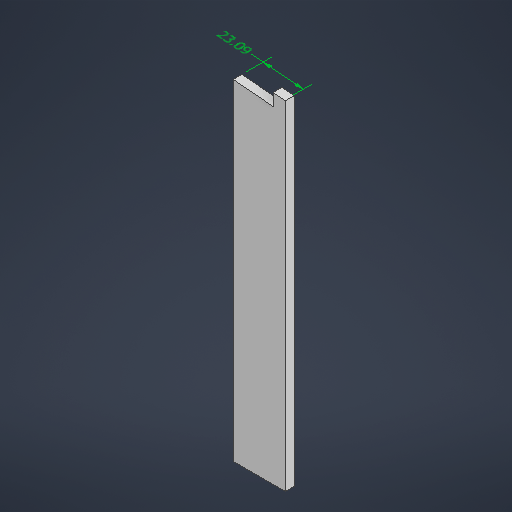
# Autodesk Inventor part: protostand
Saved by Autodesk Inventor 2026.2 (Build 302298000, 298)
## iProperties
Created: 2026-04-18
Part Number: protostand
Material: Generic
Document SubType Name: Modeling
Designer: danda
Density: 1 g/cm^3
Appearance: Default
Author: danda
Autodesk Inventor part; units mm, degrees
ref_plane "YZ Plane" through (0, 0, 0) normal (1, 0, 0) x (0, 1, 0)
ref_plane "XZ Plane" through (0, 0, 0) normal (0, 1, 0) x (-1, 0, 0)
ref_plane "XY Plane" through (0, 0, 0) normal (0, 0, 1) x (1, 0, 0)
sketch "Sketch1" plane through (0, 0, 0) normal (0, 0, 1) x (1, 0, 0)
  line L0 (65.4735, 181.5397) -> (65.4735, -8.4603)
  line L1 (65.4735, -8.4603) -> (95.4735, -8.4603)
  line L2 (95.4735, -8.4603) -> (95.4735, 178.9151)
  line L3 (65.4735, 181.5397) -> (95.4735, 178.9151)
  line L4 (65.4735, 181.5397) -> (99.7821, 181.5397) construction
  line L5 (95.4735, 178.9151) -> (95.4735, 186.5397)
  line L6 (95.4735, 186.5397) -> (88.4735, 186.5397)
  line L7 (88.4735, 186.5397) -> (88.4735, 179.5275)
  line L8 (88.4735, 186.5397) -> (98.471, 185.6651)
  line L9 (88.4735, 186.5397) -> (98.5092, 186.5397) construction
  point P0 (0, 0)
  point P1 (95.4735, 185.9273)
  dimension "d0" = 190
  dimension "d1" = 30
  dimension "d2" = 5
  dimension "d4" = 7
  dimension "d5" = 5
  dimension "d6" = 5
  constraints: 20 end point, 5 perpendicular, 2 horizontal, 1 equal length, 1 point on line, 1 vertical
  measures "d0" distance of L0.start L0.end
  measures "d1" distance of L0.end L1.end
  measures "d2" angle of L3 L4
  measures "d4" distance of L5.end L6.end
  measures "d5" distance between parallel lines of L6 L4
  measures "d6" angle of L8 L9
extrude "Extrusion1" add sketch "Sketch1" along normal blind 5 contours L3 L2 L1 L0 | L7 L8 L5 L3
body "Solid1"
